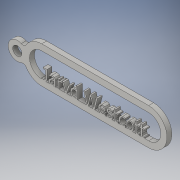
# Autodesk Inventor part: Key
Saved by Autodesk Inventor 2016 (Build 200138000, 138)
## iProperties
Created: 2017-09-07
Part Number: Key
Material: Generic
Document SubType Name: Modeling
Designer: Juan Alvarez
Density: 1 g/cm^3
Appearance: Default
Author: Juan Alvarez
Autodesk Inventor part; units mm, degrees
ref_plane "YZ Plane" through (0, 0, 0) normal (1, 0, 0) x (0, 1, 0)
ref_plane "XZ Plane" through (0, 0, 0) normal (0, 1, 0) x (-1, 0, 0)
ref_plane "XY Plane" through (0, 0, 0) normal (0, 0, 1) x (1, 0, 0)
sketch "Sketch1" plane through (0, 0, 0) normal (0, 0, 1) x (1, 0, 0)
  line L0 (-44.45, 0) -> (44.45, 0) construction
  line L1 (-44.45, -15.24) -> (44.45, -15.24)
  line L2 (44.45, 15.24) -> (-44.45, 15.24)
  arc A0 (44.45, -15.24) -> (44.45, 15.24) centre (44.45, 0) ccw
  line L3 (-44.45, 10.16) -> (44.45, 10.16)
  arc A1 (44.45, -10.16) -> (44.45, 10.16) centre (44.45, 0) ccw
  line L4 (44.45, -10.16) -> (-44.45, -10.16)
  arc A2 (-44.45, 10.16) -> (-44.45, -10.16) centre (-44.45, 0) ccw
  circle A3 centre (-64.77, 0) radius 3.81
  arc A4 (-61.4643, 6.8656) -> (-61.4643, -6.8656) centre (-64.77, 0) ccw
  arc A5 (-44.45, 15.24) -> (-57.3909, 8.0493) centre (-44.45, 0) ccw
  arc A6 (-57.3909, -8.0493) -> (-44.45, -15.24) centre (-44.45, 0) ccw
  arc A7 (-61.4643, 6.8656) -> (-57.3909, 8.0493) centre (-60.0869, 9.7263) ccw
  arc A8 (-57.3909, -8.0493) -> (-61.4643, -6.8656) centre (-60.0869, -9.7263) ccw
  point P0 (0, 0)
  point P1 (0, 0)
  dimension "d0" = 88.9
  dimension "d1" = 15.24
  dimension "d2" = 5.08
  dimension "d3" = 3.81
  dimension "d4" = 3.81
  dimension "d5" = 20.32
  dimension "d6" = 3.175
  dimension "d7" = 10.16
  dimension "d8" = 15.24
  constraints: 16 point on circle, 12 end point, 9 centre point, 8 tangent, 2 parallel, 1 coincident, 1 equal radius, 1 horizontal, 1 horizontal alignment, 1 midpoint, 2 other
  measures "d0" distance of L0.start L0.end
  measures "d1" radius of A0
  measures "d2" distance between parallel lines of L2 L3
  measures "d3" radius of A3
  measures "d4" radial gap between concentric circles of A3 A4
  measures "d5" distance of L0.start A3.centre
  measures "d6" radius of A7
  measures "d7" radius of A2
  measures "d8" radius of A5
sketch "Sketch2" plane through (0, 0, 0) normal (0, 0, 1) x (1, 0, 0)
  line L0 (-44.5962, -0.6319) -> (44.0546, -0.6319) construction
  line L1 (44.0546, -0.6319) -> (44.0546, -17.6038) construction
  line L2 (44.0546, -17.6038) -> (-44.5962, -17.6038) construction
  line L3 (-44.5962, -17.6038) -> (-44.5962, -0.6319) construction
  spline S0 degree 2 poles (-40.0422, -8.1037) (-40.0422, -9.3542) (-41.5705, -10.7127) (-42.8595, -10.7127) knots 0 0 0 1 2 2 2
  spline S1 degree 2 poles (-42.8595, -10.7127) (-43.1683, -10.7127) (-44.1949, -10.6046) (-44.5422, -10.5274) knots 0 0 0 1 2 2 2
  line L4 (-44.5422, -10.5274) -> (-44.5422, -9.3079)
  line L5 (-44.5422, -9.3079) -> (-44.4727, -9.3079)
  spline S2 degree 2 poles (-44.4727, -9.3079) (-44.2103, -9.4005) (-43.4307, -9.6166) (-43.0293, -9.6166) knots 0 0 0 1 2 2 2
  spline S3 degree 2 poles (-43.0293, -9.6166) (-42.4427, -9.6166) (-41.7403, -9.3465) (-41.5782, -9.0995) knots 0 0 0 1 2 2 2
  spline S4 degree 2 poles (-41.5782, -9.0995) (-41.4007, -8.8447) (-41.308, -8.1037) (-41.308, -7.6174) knots 0 0 0 1 2 2 2
  line L6 (-41.308, -7.6174) -> (-41.308, -2.0676)
  line L7 (-41.308, -2.0676) -> (-43.3226, -2.0676)
  line L8 (-43.3226, -2.0676) -> (-43.3226, -1.0565)
  line L9 (-43.3226, -1.0565) -> (-40.0422, -1.0565)
  line L10 (-40.0422, -1.0565) -> (-40.0422, -8.1037)
  spline S5 degree 2 poles (-34.2839, -9.825) (-34.4306, -9.9331) (-34.9246, -10.319) (-35.1562, -10.4348) knots 0 0 0 1 2 2 2
  spline S6 degree 2 poles (-35.1562, -10.4348) (-35.4726, -10.6046) (-36.067, -10.7822) (-36.6073, -10.7822) knots 0 0 0 1 2 2 2
  spline S7 degree 2 poles (-36.6073, -10.7822) (-37.0473, -10.7822) (-37.8423, -10.4502) (-38.1433, -10.1492) knots 0 0 0 1 2 2 2
  spline S8 degree 2 poles (-38.1433, -10.1492) (-38.4289, -9.8559) (-38.7763, -8.9914) (-38.7763, -8.5128) knots 0 0 0 1 2 2 2
  spline S9 degree 2 poles (-38.7763, -8.5128) (-38.7763, -7.7718) (-38.151, -6.7221) (-37.4718, -6.421) knots 0 0 0 1 2 2 2
  spline S10 degree 2 poles (-37.4718, -6.421) (-36.8697, -6.1432) (-35.2333, -5.9347) (-34.2839, -5.8807) knots 0 0 0 1 2 2 2
  line L11 (-34.2839, -5.8807) -> (-34.2839, -5.6492)
  spline S11 degree 2 poles (-34.2839, -5.6492) (-34.2839, -5.2323) (-34.5386, -4.7152) (-34.7702, -4.5685) knots 0 0 0 1 2 2 2
  spline S12 degree 2 poles (-34.7702, -4.5685) (-35.0018, -4.4219) (-35.6656, -4.3292) (-36.0207, -4.3292) knots 0 0 0 1 2 2 2
  spline S13 degree 2 poles (-36.0207, -4.3292) (-36.4375, -4.3292) (-37.5644, -4.5762) (-38.1279, -4.8155) knots 0 0 0 1 2 2 2
  line L12 (-38.1279, -4.8155) -> (-38.1974, -4.8155)
  line L13 (-38.1974, -4.8155) -> (-38.1974, -3.5882)
  spline S14 degree 2 poles (-38.1974, -3.5882) (-37.8655, -3.4956) (-36.6227, -3.264) (-36.0129, -3.264) knots 0 0 0 1 2 2 2
  spline S15 degree 2 poles (-36.0129, -3.264) (-35.2719, -3.264) (-34.2608, -3.4956) (-33.8594, -3.7966) knots 0 0 0 1 2 2 2
  spline S16 degree 2 poles (-33.8594, -3.7966) (-33.4657, -4.09) (-33.0798, -5.0239) (-33.0798, -5.6955) knots 0 0 0 1 2 2 2
  line L14 (-33.0798, -5.6955) -> (-33.0798, -10.5815)
  line L15 (-33.0798, -10.5815) -> (-34.2839, -10.5815)
  line L16 (-34.2839, -10.5815) -> (-34.2839, -9.825)
  line L17 (-34.2839, -8.8216) -> (-34.2839, -6.8378)
  spline S17 degree 2 poles (-34.2839, -6.8378) (-34.7162, -6.8764) (-36.0207, -7.0077) (-36.4298, -7.1312) knots 0 0 0 1 2 2 2
  spline S18 degree 2 poles (-36.4298, -7.1312) (-36.9083, -7.2778) (-37.5335, -7.8876) (-37.5335, -8.4279) knots 0 0 0 1 2 2 2
  spline S19 degree 2 poles (-37.5335, -8.4279) (-37.5335, -9.0454) (-36.8389, -9.6706) (-36.175, -9.6706) knots 0 0 0 1 2 2 2
  spline S20 degree 2 poles (-36.175, -9.6706) (-35.6116, -9.6706) (-34.6853, -9.1844) (-34.2839, -8.8216) knots 0 0 0 1 2 2 2
  line L18 (-27.5994, -4.7229) -> (-27.6612, -4.7229)
  spline S21 degree 2 poles (-27.6612, -4.7229) (-27.8001, -4.6843) (-28.1012, -4.6689) (-28.3096, -4.6689) knots 0 0 0 1 2 2 2
  spline S22 degree 2 poles (-28.3096, -4.6689) (-28.7959, -4.6689) (-29.753, -5.0934) (-30.1852, -5.5102) knots 0 0 0 1 2 2 2
  line L19 (-30.1852, -5.5102) -> (-30.1852, -10.5815)
  line L20 (-30.1852, -10.5815) -> (-31.3894, -10.5815)
  line L21 (-31.3894, -10.5815) -> (-31.3894, -3.4339)
  line L22 (-31.3894, -3.4339) -> (-30.1852, -3.4339)
  line L23 (-30.1852, -3.4339) -> (-30.1852, -4.499)
  spline S23 degree 2 poles (-30.1852, -4.499) (-29.5291, -3.9124) (-28.5489, -3.4339) (-28.0857, -3.4339) knots 0 0 0 1 2 2 2
  spline S24 degree 2 poles (-28.0857, -3.4339) (-27.9005, -3.4339) (-27.7152, -3.4493) (-27.5994, -3.4724) knots 0 0 0 1 2 2 2
  line L24 (-27.5994, -3.4724) -> (-27.5994, -4.7229)
  line L25 (-21.0539, -3.4339) -> (-24.8979, -13.2136)
  line L26 (-24.8979, -13.2136) -> (-26.1869, -13.2136)
  line L27 (-26.1869, -13.2136) -> (-24.9056, -10.2341)
  line L28 (-24.9056, -10.2341) -> (-27.4991, -3.4339)
  line L29 (-27.4991, -3.4339) -> (-26.2023, -3.4339)
  line L30 (-26.2023, -3.4339) -> (-24.2495, -8.729)
  line L31 (-24.2495, -8.729) -> (-22.3044, -3.4339)
  line L32 (-22.3044, -3.4339) -> (-21.0539, -3.4339)
  line L33 (-14.6473, -10.5815) -> (-15.8514, -10.5815)
  line L34 (-15.8514, -10.5815) -> (-15.8514, -9.8559)
  spline S25 degree 2 poles (-15.8514, -9.8559) (-16.1293, -10.0875) (-16.5384, -10.3962) (-16.8163, -10.5274) knots 0 0 0 1 2 2 2
  spline S26 degree 2 poles (-16.8163, -10.5274) (-17.071, -10.6509) (-17.619, -10.7822) (-17.9818, -10.7822) knots 0 0 0 1 2 2 2
  spline S27 degree 2 poles (-17.9818, -10.7822) (-18.5685, -10.7822) (-19.5565, -10.2959) (-19.9038, -9.825) knots 0 0 0 1 2 2 2
  spline S28 degree 2 poles (-19.9038, -9.825) (-20.2511, -9.3542) (-20.6371, -7.9648) (-20.6371, -7.0617) knots 0 0 0 1 2 2 2
  spline S29 degree 2 poles (-20.6371, -7.0617) (-20.6371, -6.12) (-20.1508, -4.7461) (-19.7263, -4.2289) knots 0 0 0 1 2 2 2
  spline S30 degree 2 poles (-19.7263, -4.2289) (-19.3326, -3.7658) (-18.2288, -3.2332) (-17.619, -3.2332) knots 0 0 0 1 2 2 2
  spline S31 degree 2 poles (-17.619, -3.2332) (-17.0864, -3.2332) (-16.2914, -3.4724) (-15.8514, -3.7195) knots 0 0 0 1 2 2 2
  line L35 (-15.8514, -3.7195) -> (-15.8514, -0.6319)
  line L36 (-15.8514, -0.6319) -> (-14.6473, -0.6319)
  line L37 (-14.6473, -0.6319) -> (-14.6473, -10.5815)
  line L38 (-15.8514, -8.8447) -> (-15.8514, -4.7152)
  spline S32 degree 2 poles (-15.8514, -4.7152) (-16.2991, -4.499) (-17.0093, -4.337) (-17.4183, -4.337) knots 0 0 0 1 2 2 2
  spline S33 degree 2 poles (-17.4183, -4.337) (-18.3446, -4.337) (-19.3944, -5.7263) (-19.3944, -7.0385) knots 0 0 0 1 2 2 2
  spline S34 degree 2 poles (-19.3944, -7.0385) (-19.3944, -8.3044) (-18.5916, -9.6398) (-17.7039, -9.6398) knots 0 0 0 1 2 2 2
  spline S35 degree 2 poles (-17.7039, -9.6398) (-17.2331, -9.6398) (-16.276, -9.2075) (-15.8514, -8.8447) knots 0 0 0 1 2 2 2
  line L39 (1.9558, -1.0565) -> (-0.437, -10.5815)
  line L40 (-0.437, -10.5815) -> (-1.8572, -10.5815)
  line L41 (-1.8572, -10.5815) -> (-3.7947, -2.6774)
  line L42 (-3.7947, -2.6774) -> (-5.6781, -10.5815)
  line L43 (-5.6781, -10.5815) -> (-7.0829, -10.5815)
  line L44 (-7.0829, -10.5815) -> (-9.5143, -1.0565)
  line L45 (-9.5143, -1.0565) -> (-8.2098, -1.0565)
  line L46 (-8.2098, -1.0565) -> (-6.2956, -8.9528)
  line L47 (-6.2956, -8.9528) -> (-4.3967, -1.0565)
  line L48 (-4.3967, -1.0565) -> (-3.1077, -1.0565)
  line L49 (-3.1077, -1.0565) -> (-1.1934, -9.0454)
  line L50 (-1.1934, -9.0454) -> (0.7131, -1.0565)
  line L51 (0.7131, -1.0565) -> (1.9558, -1.0565)
  spline S36 degree 2 poles (6.1008, -10.7436) (4.3873, -10.7436) (2.5039, -8.8216) (2.5039, -7.0463) knots 0 0 0 1 2 2 2
  spline S37 degree 2 poles (2.5039, -7.0463) (2.5039, -5.3018) (4.3332, -3.2332) (5.8075, -3.2332) knots 0 0 0 1 2 2 2
  spline S38 degree 2 poles (5.8075, -3.2332) (6.4713, -3.2332) (7.4979, -3.6191) (7.8762, -4.0282) knots 0 0 0 1 2 2 2
  spline S39 degree 2 poles (7.8762, -4.0282) (8.2621, -4.4373) (8.6712, -5.6183) (8.6712, -6.4751) knots 0 0 0 1 2 2 2
  line L52 (8.6712, -6.4751) -> (8.6712, -7.1312)
  line L53 (8.6712, -7.1312) -> (3.7234, -7.1312)
  spline S40 degree 2 poles (3.7234, -7.1312) (3.7234, -8.3739) (4.9739, -9.6938) (6.0854, -9.6938) knots 0 0 0 1 2 2 2
  spline S41 degree 2 poles (6.0854, -9.6938) (6.4791, -9.6938) (7.2432, -9.5163) (7.552, -9.3773) knots 0 0 0 1 2 2 2
  spline S42 degree 2 poles (7.552, -9.3773) (7.8762, -9.223) (8.3239, -8.9528) (8.4705, -8.8293) knots 0 0 0 1 2 2 2
  line L54 (8.4705, -8.8293) -> (8.54, -8.8293)
  line L55 (8.54, -8.8293) -> (8.54, -10.1415)
  spline S43 degree 2 poles (8.54, -10.1415) (8.3316, -10.2264) (7.6986, -10.4734) (7.4516, -10.5429) knots 0 0 0 1 2 2 2
  spline S44 degree 2 poles (7.4516, -10.5429) (7.1043, -10.6432) (6.5331, -10.7436) (6.1008, -10.7436) knots 0 0 0 1 2 2 2
  spline S45 degree 2 poles (7.4979, -6.2126) (7.4825, -5.7263) (7.2818, -5.0162) (7.0888, -4.7769) knots 0 0 0 1 2 2 2
  spline S46 degree 2 poles (7.0888, -4.7769) (6.8804, -4.5068) (6.2243, -4.2212) (5.7381, -4.2212) knots 0 0 0 1 2 2 2
  spline S47 degree 2 poles (5.7381, -4.2212) (5.2595, -4.2212) (4.588, -4.5068) (4.3101, -4.7846) knots 0 0 0 1 2 2 2
  spline S48 degree 2 poles (4.3101, -4.7846) (4.0399, -5.0702) (3.762, -5.7572) (3.7234, -6.2126) knots 0 0 0 1 2 2 2
  line L56 (3.7234, -6.2126) -> (7.4979, -6.2126)
  spline S49 degree 2 poles (11.8205, -10.7513) (11.1026, -10.7513) (9.8599, -10.3653) (9.4508, -10.1492) knots 0 0 0 1 2 2 2
  line L57 (9.4508, -10.1492) -> (9.4508, -8.7984)
  line L58 (9.4508, -8.7984) -> (9.5125, -8.7984)
  spline S50 degree 2 poles (9.5125, -8.7984) (9.6669, -8.9219) (10.0837, -9.2152) (10.4311, -9.3773) knots 0 0 0 1 2 2 2
  spline S51 degree 2 poles (10.4311, -9.3773) (10.7321, -9.524) (11.4731, -9.7401) (11.8668, -9.7401) knots 0 0 0 1 2 2 2
  spline S52 degree 2 poles (11.8668, -9.7401) (12.1524, -9.7401) (12.8085, -9.6089) (12.9628, -9.5008) knots 0 0 0 1 2 2 2
  spline S53 degree 2 poles (12.9628, -9.5008) (13.1867, -9.3542) (13.3874, -9.0223) (13.3874, -8.6826) knots 0 0 0 1 2 2 2
  spline S54 degree 2 poles (13.3874, -8.6826) (13.3874, -8.2581) (12.9243, -7.8181) (12.3299, -7.6715) knots 0 0 0 1 2 2 2
  spline S55 degree 2 poles (12.3299, -7.6715) (12.0983, -7.6174) (11.3573, -7.4631) (11.0409, -7.3782) knots 0 0 0 1 2 2 2
  spline S56 degree 2 poles (11.0409, -7.3782) (10.2227, -7.1389) (9.4817, -6.1509) (9.4817, -5.4485) knots 0 0 0 1 2 2 2
  spline S57 degree 2 poles (9.4817, -5.4485) (9.4817, -4.4759) (10.9405, -3.264) (12.1447, -3.264) knots 0 0 0 1 2 2 2
  spline S58 degree 2 poles (12.1447, -3.264) (12.739, -3.264) (13.9431, -3.5574) (14.3522, -3.7812) knots 0 0 0 1 2 2 2
  line L59 (14.3522, -3.7812) -> (14.3522, -5.0702)
  line L60 (14.3522, -5.0702) -> (14.2905, -5.0702)
  spline S59 degree 2 poles (14.2905, -5.0702) (13.8274, -4.6997) (12.7004, -4.2752) (12.1215, -4.2752) knots 0 0 0 1 2 2 2
  spline S60 degree 2 poles (12.1215, -4.2752) (11.5272, -4.2752) (10.709, -4.7769) (10.709, -5.2786) knots 0 0 0 1 2 2 2
  spline S61 degree 2 poles (10.709, -5.2786) (10.709, -5.7341) (11.1952, -6.174) (11.7356, -6.313) knots 0 0 0 1 2 2 2
  spline S62 degree 2 poles (11.7356, -6.313) (11.998, -6.3824) (12.6618, -6.5214) (13.0246, -6.6063) knots 0 0 0 1 2 2 2
  spline S63 degree 2 poles (13.0246, -6.6063) (13.8119, -6.807) (14.6147, -7.7255) (14.6147, -8.5205) knots 0 0 0 1 2 2 2
  spline S64 degree 2 poles (14.6147, -8.5205) (14.6147, -8.9837) (14.2519, -9.8019) (13.8968, -10.1029) knots 0 0 0 1 2 2 2
  spline S65 degree 2 poles (13.8968, -10.1029) (13.5186, -10.4194) (12.5538, -10.7513) (11.8205, -10.7513) knots 0 0 0 1 2 2 2
  spline S66 degree 2 poles (17.8952, -10.7204) (16.9149, -10.7204) (15.8111, -9.6012) (15.8111, -8.3893) knots 0 0 0 1 2 2 2
  line L61 (15.8111, -8.3893) -> (15.8111, -4.4296)
  line L62 (15.8111, -4.4296) -> (15.0006, -4.4296)
  line L63 (15.0006, -4.4296) -> (15.0006, -3.4339)
  line L64 (15.0006, -3.4339) -> (15.8111, -3.4339)
  line L65 (15.8111, -3.4339) -> (15.8111, -1.3807)
  line L66 (15.8111, -1.3807) -> (17.0152, -1.3807)
  line L67 (17.0152, -1.3807) -> (17.0152, -3.4339)
  line L68 (17.0152, -3.4339) -> (19.2305, -3.4339)
  line L69 (19.2305, -3.4339) -> (19.2305, -4.4296)
  line L70 (19.2305, -4.4296) -> (17.0152, -4.4296)
  line L71 (17.0152, -4.4296) -> (17.0152, -7.8336)
  spline S67 degree 2 poles (17.0152, -7.8336) (17.0152, -8.3739) (17.0538, -8.9682) (17.185, -9.223) knots 0 0 0 1 2 2 2
  spline S68 degree 2 poles (17.185, -9.223) (17.2931, -9.4468) (17.7794, -9.6706) (18.1962, -9.6706) knots 0 0 0 1 2 2 2
  spline S69 degree 2 poles (18.1962, -9.6706) (18.4895, -9.6706) (19.0375, -9.4931) (19.161, -9.4391) knots 0 0 0 1 2 2 2
  line L72 (19.161, -9.4391) -> (19.2305, -9.4391)
  line L73 (19.2305, -9.4391) -> (19.2305, -10.5197)
  spline S70 degree 2 poles (19.2305, -10.5197) (18.8909, -10.6123) (18.1962, -10.7204) (17.8952, -10.7204) knots 0 0 0 1 2 2 2
  spline S71 degree 2 poles (22.9587, -10.7436) (22.2177, -10.7436) (20.9904, -10.2881) (20.5504, -9.825) knots 0 0 0 1 2 2 2
  spline S72 degree 2 poles (20.5504, -9.825) (20.1105, -9.3696) (19.6242, -7.9648) (19.6242, -7.0231) knots 0 0 0 1 2 2 2
  spline S73 degree 2 poles (19.6242, -7.0231) (19.6242, -6.0814) (20.1259, -4.7075) (20.5504, -4.2443) knots 0 0 0 1 2 2 2
  spline S74 degree 2 poles (20.5504, -4.2443) (20.975, -3.7735) (22.2331, -3.2718) (22.9587, -3.2718) knots 0 0 0 1 2 2 2
  spline S75 degree 2 poles (22.9587, -3.2718) (23.5453, -3.2718) (24.6414, -3.6037) (25.0659, -3.8198) knots 0 0 0 1 2 2 2
  line L74 (25.0659, -3.8198) -> (25.0659, -5.1706)
  line L75 (25.0659, -5.1706) -> (24.9965, -5.1706)
  spline S76 degree 2 poles (24.9965, -5.1706) (24.8652, -5.0625) (24.4639, -4.7846) (24.1783, -4.638) knots 0 0 0 1 2 2 2
  spline S77 degree 2 poles (24.1783, -4.638) (23.9235, -4.5145) (23.2443, -4.3215) (22.9355, -4.3215) knots 0 0 0 1 2 2 2
  spline S78 degree 2 poles (22.9355, -4.3215) (22.0016, -4.3215) (20.8669, -5.7341) (20.8669, -7.0231) knots 0 0 0 1 2 2 2
  spline S79 degree 2 poles (20.8669, -7.0231) (20.8669, -8.2813) (21.963, -9.6938) (22.9355, -9.6938) knots 0 0 0 1 2 2 2
  spline S80 degree 2 poles (22.9355, -9.6938) (23.5222, -9.6938) (24.5874, -9.2075) (24.9965, -8.8293) knots 0 0 0 1 2 2 2
  line L76 (24.9965, -8.8293) -> (25.0659, -8.8293)
  line L77 (25.0659, -8.8293) -> (25.0659, -10.1801)
  spline S81 degree 2 poles (25.0659, -10.1801) (24.8884, -10.265) (24.3481, -10.5043) (24.132, -10.5583) knots 0 0 0 1 2 2 2
  spline S82 degree 2 poles (24.132, -10.5583) (23.8232, -10.6509) (23.3369, -10.7436) (22.9587, -10.7436) knots 0 0 0 1 2 2 2
  spline S83 degree 2 poles (32.036, -7.0077) (32.036, -8.8139) (30.2993, -10.7822) (28.8481, -10.7822) knots 0 0 0 1 2 2 2
  spline S84 degree 2 poles (28.8481, -10.7822) (27.3584, -10.7822) (25.6526, -8.7521) (25.6526, -7.0077) knots 0 0 0 1 2 2 2
  spline S85 degree 2 poles (25.6526, -7.0077) (25.6526, -5.2169) (27.4124, -3.2332) (28.8481, -3.2332) knots 0 0 0 1 2 2 2
  spline S86 degree 2 poles (28.8481, -3.2332) (30.2993, -3.2332) (32.036, -5.2092) (32.036, -7.0077) knots 0 0 0 1 2 2 2
  spline S87 degree 2 poles (30.7933, -7.0077) (30.7933, -5.6183) (29.7821, -4.2675) (28.8481, -4.2675) knots 0 0 0 1 2 2 2
  spline S88 degree 2 poles (28.8481, -4.2675) (27.9142, -4.2675) (26.8953, -5.6183) (26.8953, -7.0077) knots 0 0 0 1 2 2 2
  spline S89 degree 2 poles (26.8953, -7.0077) (26.8953, -8.3584) (27.9142, -9.7478) (28.8481, -9.7478) knots 0 0 0 1 2 2 2
  spline S90 degree 2 poles (28.8481, -9.7478) (29.7744, -9.7478) (30.7933, -8.3816) (30.7933, -7.0077) knots 0 0 0 1 2 2 2
  spline S91 degree 2 poles (35.4323, -10.7204) (34.452, -10.7204) (33.3482, -9.6012) (33.3482, -8.3893) knots 0 0 0 1 2 2 2
  line L78 (33.3482, -8.3893) -> (33.3482, -4.4296)
  line L79 (33.3482, -4.4296) -> (32.5377, -4.4296)
  line L80 (32.5377, -4.4296) -> (32.5377, -3.4339)
  line L81 (32.5377, -3.4339) -> (33.3482, -3.4339)
  line L82 (33.3482, -3.4339) -> (33.3482, -1.3807)
  line L83 (33.3482, -1.3807) -> (34.5523, -1.3807)
  line L84 (34.5523, -1.3807) -> (34.5523, -3.4339)
  line L85 (34.5523, -3.4339) -> (36.7676, -3.4339)
  line L86 (36.7676, -3.4339) -> (36.7676, -4.4296)
  line L87 (36.7676, -4.4296) -> (34.5523, -4.4296)
  line L88 (34.5523, -4.4296) -> (34.5523, -7.8336)
  spline S92 degree 2 poles (34.5523, -7.8336) (34.5523, -8.3739) (34.5909, -8.9682) (34.7221, -9.223) knots 0 0 0 1 2 2 2
  spline S93 degree 2 poles (34.7221, -9.223) (34.8302, -9.4468) (35.3165, -9.6706) (35.7333, -9.6706) knots 0 0 0 1 2 2 2
  spline S94 degree 2 poles (35.7333, -9.6706) (36.0266, -9.6706) (36.5747, -9.4931) (36.6982, -9.4391) knots 0 0 0 1 2 2 2
  line L89 (36.6982, -9.4391) -> (36.7676, -9.4391)
  line L90 (36.7676, -9.4391) -> (36.7676, -10.5197)
  spline S95 degree 2 poles (36.7676, -10.5197) (36.428, -10.6123) (35.7333, -10.7204) (35.4323, -10.7204) knots 0 0 0 1 2 2 2
  spline S96 degree 2 poles (39.8166, -10.7204) (38.8363, -10.7204) (37.7325, -9.6012) (37.7325, -8.3893) knots 0 0 0 1 2 2 2
  line L91 (37.7325, -8.3893) -> (37.7325, -4.4296)
  line L92 (37.7325, -4.4296) -> (36.922, -4.4296)
  line L93 (36.922, -4.4296) -> (36.922, -3.4339)
  line L94 (36.922, -3.4339) -> (37.7325, -3.4339)
  line L95 (37.7325, -3.4339) -> (37.7325, -1.3807)
  line L96 (37.7325, -1.3807) -> (38.9366, -1.3807)
  line L97 (38.9366, -1.3807) -> (38.9366, -3.4339)
  line L98 (38.9366, -3.4339) -> (41.1519, -3.4339)
  line L99 (41.1519, -3.4339) -> (41.1519, -4.4296)
  line L100 (41.1519, -4.4296) -> (38.9366, -4.4296)
  line L101 (38.9366, -4.4296) -> (38.9366, -7.8336)
  spline S97 degree 2 poles (38.9366, -7.8336) (38.9366, -8.3739) (38.9752, -8.9682) (39.1064, -9.223) knots 0 0 0 1 2 2 2
  spline S98 degree 2 poles (39.1064, -9.223) (39.2145, -9.4468) (39.7008, -9.6706) (40.1176, -9.6706) knots 0 0 0 1 2 2 2
  spline S99 degree 2 poles (40.1176, -9.6706) (40.4109, -9.6706) (40.9589, -9.4931) (41.0824, -9.4391) knots 0 0 0 1 2 2 2
  line L102 (41.0824, -9.4391) -> (41.1519, -9.4391)
  line L103 (41.1519, -9.4391) -> (41.1519, -10.5197)
  spline S100 degree 2 poles (41.1519, -10.5197) (40.8123, -10.6123) (40.1176, -10.7204) (39.8166, -10.7204) knots 0 0 0 1 2 2 2
  point P0 (0, 0)
  constraints: 2 other
extrude "Extrusion1" add sketch "Sketch2" along normal blind 4.064
extrude "Extrusion2" add sketch "Sketch1" along normal blind 4.064
body "Solid1"
